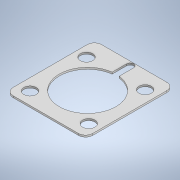
# Autodesk Inventor part: cylinder head gasket
Saved by Autodesk Inventor 2020 (Build 240168000, 168)
## iProperties
Created: 2020-08-05
Part Number: cylinder head gasket
Material: Generic
Document SubType Name: Modeling
Designer: benny
Density: 1 g/cm^3
Appearance: Default
Author: benny
Autodesk Inventor part; units mm, degrees
ref_plane "YZ Plane" through (0, 0, 0) normal (1, 0, 0) x (0, 1, 0)
ref_plane "XZ Plane" through (0, 0, 0) normal (0, 1, 0) x (-1, 0, 0)
ref_plane "XY Plane" through (0, 0, 0) normal (0, 0, 1) x (1, 0, 0)
sketch "Sketch1" plane through (0, 0, 0) normal (0, 1, 0) x (-1, 0, 0)
  line L0 (-22.5, 23.6526) -> (22.5, 23.6526)
  line L1 (22.5, 23.6526) -> (22.5, -26.3474)
  line L2 (22.5, -26.3474) -> (-22.5, -26.3474)
  line L3 (-22.5, -26.3474) -> (-22.5, 23.6526)
  line L4 (-22.5, 23.6526) -> (22.5, -26.3474) construction
  line L5 (22.5, 23.6526) -> (-22.5, -26.3474) construction
  point P0 (0, 0)
  point P1 (0, -1.3474)
  dimension "d0" = 45
  dimension "d1" = 50
  constraints: 12 end point, 2 midpoint, 2 parallel, 1 horizontal, 1 perpendicular
  measures "d0" distance of L1.end L2.end
  measures "d1" distance of L0.end L1.end
extrude "Extrusion1" add sketch "Sketch1" along normal blind 1
fillet "Fillet1" radius 4 4 edges at (22.5, 0.5, 23.6526) (-22.5, 0.5, 23.6526) (-22.5, 0.5, -26.3474) (22.5, 0.5, -26.3474)
sketch "Sketch2" plane through (0, 1, 0) normal (0, 1, 0) x (1, 0, 0)
  circle A0 centre (0, 0) radius 16
  dimension "d5" = 32
  constraints: 1 centre point, 1 coincident
  measures "d5" diameter of A0
extrude "Extrusion2" cut sketch "Sketch2" against normal blind 1
sketch "Sketch3" plane through (0, 1, 0) normal (0, 1, 0) x (1, 0, 0)
  line L0 (0, 0) -> (-15.9515, -16.5696)
  circle A0 centre (-15.9515, -16.5696) radius 3.5
  dimension "d8" = 23
  dimension "d9" = 7
  constraints: 2 end point, 1 centre point, 1 coincident
  measures "d8" distance of L0.start L0.end
  measures "d9" diameter of A0
extrude "Extrusion3" cut sketch "Sketch3" against normal blind 1
pattern_circular "Circular Pattern1" count 4 over 360 about axis through (0, 1, 0) along (0, -1, 0) of "Extrusion3"
sketch "Sketch4" plane through (0, 1, 0) normal (0, 1, 0) x (1, 0, 0)
  line L0 (0, 0) -> (0, 24)
  circle A0 centre (0, 24) radius 2
  dimension "d15" = 24
  dimension "d16" = 4
  constraints: 2 end point, 1 centre point, 1 coincident, 1 vertical
  measures "d15" distance of L0.start L0.end
  measures "d16" diameter of A0
extrude "Extrusion4" cut sketch "Sketch4" against normal blind 1
sketch "Sketch5" plane through (0, 1, 0) normal (0, 1, 0) x (1, 0, 0)
  circle A0 centre (0, 24) radius 2 projected
  line L0 (-2, 8) -> (2, 8)
  line L1 (2, 8) -> (2, 24)
  line L2 (2, 24) -> (-2, 24)
  line L3 (-2, 24) -> (-2, 8)
  circle A1 centre (0, 0) radius 16 projected
  line L4 (-2, 8) -> (2, 24) construction
  line L5 (2, 8) -> (-2, 24) construction
  point P0 (0, 16)
  constraints: 12 end point, 2 midpoint, 2 parallel, 1 horizontal, 1 perpendicular, 1 vertical alignment, 3 other
extrude "Extrusion5" cut sketch "Sketch5" against normal blind 1 contours L1 A1 L3 A0 | L1 L0 L3 A1 picked at (-0.2227, 10.662)
body "Solid1"
